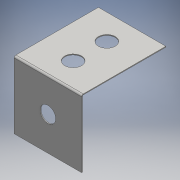
# Autodesk Inventor part: L Braket for Wheels
Saved by Autodesk Inventor 2016 (Build 200138000, 138)
## iProperties
Created: 2017-11-07
Part Number: L Braket for Wheels
Material: Generic
Document SubType Name: Sheet Metal
Designer: M227562
Density: 1 g/cm^3
Sheet Metal Rule: Default_mm
Appearance: Default
Author: M227562
Autodesk Inventor part; units mm, degrees
ref_plane "YZ Plane" through (0, 0, 0) normal (1, 0, 0) x (0, 1, 0)
ref_plane "XZ Plane" through (0, 0, 0) normal (0, 1, 0) x (-1, 0, 0)
ref_plane "XY Plane" through (0, 0, 0) normal (0, 0, 1) x (1, 0, 0)
sketch "Sketch1" plane through (0, 0, 0) normal (0, 1, 0) x (-1, 0, 0)
  line L0 (-20, -20) -> (20, -20)
  line L1 (20, -20) -> (20, 20)
  line L2 (20, 20) -> (-20, 20)
  line L3 (-20, 20) -> (-20, -20)
  line L4 (-20, -20) -> (20, 20) construction
  line L5 (20, -20) -> (-20, 20) construction
  point P0 (0, 0)
  dimension "d0" = 40
  dimension "d1" = 40
  measures "d0" distance of L2.end L1.end
  measures "d1" distance of L1.end L0.end
extrude "Plate1" add sketch "Sketch1" along normal blind 0.5
sketch "Sketch2" plane through (20, 0, 19.5) normal (0, 0, 1) x (1, 0, 0)
  line L0 (-40, 0) -> (0, 0)
  line L1 (0, 0) -> (0, 50)
  line L2 (0, 50) -> (-40, 50)
  line L3 (-40, 50) -> (-40, 0)
  constraints: 6 end point, 1 horizontal, 1 perpendicular, 1 vertical
edge flange "Flange1" height 50 angle 90 thickness 0.5 bend radius 0.5 thickness toward (0, 0, 1) relief tear relief width 0.5 relief depth 0.25 edges at (0, 0.5, 20) wall of the first edge with corners at (-20, 0, 19.5) (20, 0, 19.5) (20, 50, 19.5) (-20, 50, 19.5)
bend "Bend1"
corner "Corner1"
sketch "Sketch3" plane through (20, 50, 19.5) normal (0, 0, -1) x (-1, 0, 0)
  line L0 (40, 0) -> (0, 0) construction
  line L1 (20, 0) -> (20, -49) construction
  line L2 (0, -49) -> (40, -49) construction
  line L3 (0, 0) -> (0, -20) construction
  line L4 (0, 0) -> (0, -49) construction
  line L5 (0, -20) -> (0, -40) construction
  line L6 (40, 0) -> (40, -49) construction
  line L7 (0, 0) -> (1.6205, 0)
  line L8 (0, 0) -> (0, -15) construction
  line L9 (0, -15) -> (20, -15) construction
  circle A0 centre (20, -15) radius 5 construction
  line L10 (0, -15) -> (0, -35) construction
  line L11 (0, -35) -> (20, -35) construction
  circle A1 centre (20, -35) radius 5 construction
  point P0 (20, -50)
  dimension "d15" = 15
  dimension "d16" = 20
  constraints: 16 end point, 7 point on line, 2 centre point, 2 coincident, 2 midpoint, 2 perpendicular
  measures "d15" distance of L0.end L8.end
  measures "d16" distance of L8.end L10.end
hole "Hole1" at (0, 35, 19.5) at (0, 15, 19.5) direction (0, 0, 1) diameter 10 end through all
sketch "Sketch4" plane through (0, 0.5, 0) normal (0, 1, 0) x (1, 0, 0)
  point P0 (0, 0)
hole "Hole2" at (0, 0.5, 0) direction (0, -1, 0) diameter 9.254 end through all
equation "\"d22\" = Thickness"
equation "\"d29\" = Thickness"
equation "\"d3\" = BendReliefWidth"
equation "\"d4\" = BendReliefDepth"
equation "\"d5\" = MinimumRemnant"
equation "\"d6\" = BendRadius"
equation "\"d9\" = BendRadius"
equation "\"d10\" = CornerReliefSize"
equation "\"d11\" = GapSize"
equation "\"d12\" = JacobiRadiusSize"
equation "\"BendRadius\" = Thickness"
equation "\"BendReliefWidth\" = Thickness"
equation "\"BendReliefDepth\" = 0.5 * Thickness"
equation "\"CornerReliefSize\" = 4 * Thickness"
equation "\"MinimumRemnant\" = 2 * Thickness"
equation "\"TransitionRadius\" = BendRadius"
equation "\"JacobiRadiusSize\" = BendRadius"
equation "\"GapSize\" = Thickness"
equation "\"d2\" = BendRadius"
equation "\"Thickness\" = 0.5"
body "Solid1"
